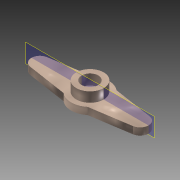
# Autodesk Inventor part: MG996RHorn
Saved by Autodesk Inventor 2014 SP1 (Build 180222100, 222)
## iProperties
Created: 2017-01-17
Part Number: MG996RHorn
Material: Generic
Document SubType Name: Modeling
Designer: danielsikar
Density: 1 g/cm^3
Appearance: Exterior - Beige
Author: danielsikar
Autodesk Inventor part; units mm, degrees
ref_plane "YZ Plane" through (0, 0, 0) normal (1, 0, 0) x (0, 1, 0)
ref_plane "XY Plane" through (0, 0, 0) normal (0, 0, 1) x (1, 0, 0)
sketch "Sketch1" plane through (0, 0, 0) normal (0, 0, 1) x (1, 0, 0)
  arc A0 (-16.6686, 2.7179) -> (-16.6686, -2.7179) centre (-16.25, 0) ccw
  arc A1 (16.6686, -2.7179) -> (16.6686, 2.7179) centre (16.25, 0) ccw
  line L0 (-3.9085, 4.6833) -> (-16.6686, 2.7179)
  line L1 (-3.9085, -4.6833) -> (-16.6686, -2.7179)
  line L2 (3.9085, -4.6833) -> (16.6686, -2.7179)
  line L3 (3.9085, 4.6833) -> (16.6686, 2.7179)
  arc A2 (-3.9085, -4.6833) -> (3.9085, -4.6833) centre (0, 0) ccw
  arc A3 (3.9085, 4.6833) -> (-3.9085, 4.6833) centre (0, 0) ccw
  point P0 (0, 4.6833)
  dimension "d2" = 5.5
  dimension "d3" = 5.5
  constraints: 8 end point, 8 point on circle, 4 centre point, 4 tangent, 1 coincident, 1 vertical alignment
  measures "d2" diameter of A0
  measures "d3" diameter of A1
extrude "Extrusion1" add sketch "Sketch1" along normal blind 2.3
sketch "Sketch2" plane through (0, 0, 2.3) normal (0, 0, 1) x (1, 0, 0)
  arc A0 (-3.9085, -4.6833) -> (3.9085, -4.6833) centre (0, 0) ccw projected
  circle A1 centre (0, 0) radius 4.45
  dimension "d6" = 8.9
  constraints: 1 centre point, 1 coincident
  measures "d6" diameter of A1
extrude "Extrusion2" add sketch "Sketch2" along normal blind 3.2
sketch "Sketch3" plane through (0, 0, 5.5) normal (0, 0, 1) x (1, 0, 0)
  circle A0 centre (0, 0) radius 4.45 projected
  circle A1 centre (0, 0) radius 2.7
  dimension "d9" = 5.4
  constraints: 1 centre point, 1 coincident
  measures "d9" diameter of A1
extrude "Extrusion3" cut sketch "Sketch3" against normal blind 3.4 contours A1
sketch "Sketch4" plane through (0, 0, 2.1) normal (0, 0, 1) x (1, 0, 0)
  circle A0 centre (0, 0) radius 2.7 projected
  circle A1 centre (0, 0) radius 1.4
  dimension "d12" = 2.8
  constraints: 1 centre point, 1 coincident
  measures "d12" diameter of A1
extrude "Extrusion4" cut sketch "Sketch4" against normal blind 3.4 contours A1
ref_plane "ConstraintPlane" through (0, 0, 0) normal (0, 1, 0) x (-1, 0, 0)
body "Solid1"
